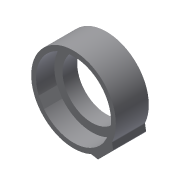
# Autodesk Inventor part: cellSTORM_objective_thread
Saved by Autodesk Inventor 2019 (Build 230136000, 136)
## iProperties
Created: 2019-10-25
Part Number: cellSTORM_objective_thread
Material: Generic
Document SubType Name: Modeling
Designer: marsikovabarbora
Density: 1 g/cm^3
Appearance: Default
Author: marsikovabarbora
Autodesk Inventor part; units mm, degrees
ref_plane "YZ Plane" through (0, 0, 0) normal (1, 0, 0) x (0, 1, 0)
ref_plane "XZ Plane" through (0, 0, 0) normal (0, 1, 0) x (-1, 0, 0)
ref_plane "XY Plane" through (0, 0, 0) normal (0, 0, 1) x (1, 0, 0)
sketch "Sketch1" plane through (0, 0, 0) normal (0, 0, 1) x (1, 0, 0)
  line L0 (9.6801, -14.008) -> (7.2052, -11.5331) construction
  line L1 (7.2052, -11.5331) -> (11.5893, -7.1491) construction
  line L2 (11.5893, -7.1491) -> (14.0642, -9.6239) construction
  line L3 (14.0642, -9.6239) -> (9.6801, -14.008) construction
  arc A0 (12.6369, -4.7496) -> (4.7496, -12.6369) centre (0, 0) ccw construction
  line L4 (10.9298, -3.0424) -> (12.6369, -4.7496) construction
  line L5 (11.6618, -4.6122) -> (10.9298, -3.0424) construction
  arc A1 (11.6618, -4.6122) -> (10.8551, -4.47) centre (11.2086, -4.8235) ccw construction
  line L6 (10.7915, -4.5335) -> (10.8551, -4.47) construction
  arc A2 (10.7915, -4.5335) -> (10.6527, -4.9738) centre (11.1451, -4.887) ccw construction
  line L7 (10.915, -6.4612) -> (10.6527, -4.9738) construction
  arc A3 (10.7761, -6.9016) -> (10.915, -6.4612) centre (10.4226, -6.548) ccw construction
  line L8 (6.9016, -10.7761) -> (10.7761, -6.9016) construction
  arc A4 (6.4612, -10.915) -> (6.9016, -10.7761) centre (6.548, -10.4226) ccw construction
  line L9 (6.4612, -10.915) -> (4.9738, -10.6527) construction
  arc A5 (4.9738, -10.6527) -> (4.5335, -10.7915) centre (4.887, -11.1451) ccw construction
  line L10 (4.5335, -10.7915) -> (4.47, -10.8551) construction
  arc A6 (4.47, -10.8551) -> (4.6122, -11.6618) centre (4.8235, -11.2086) ccw construction
  line L11 (4.6122, -11.6618) -> (3.0424, -10.9298) construction
  line L12 (3.0424, -10.9298) -> (4.7496, -12.6369) construction
  line L13 (-1.7167, -14.6498) -> (-1.7167, -17.5) construction
  line L14 (-1.7167, -17.5) -> (1.7167, -17.5) construction
  line L15 (1.7167, -14.6498) -> (1.7167, -17.5) construction
  arc A7 (1.7167, -14.6498) -> (6.9595, -13.0049) centre (0, 0) ccw construction
  arc A8 (6.9595, -13.0049) -> (8.2728, -15.1789) centre (8.2994, -13.6792) ccw construction
  line L16 (8.2728, -15.1789) -> (7.6816, -15.1684) construction
  arc A9 (8.5249, -17.8901) -> (7.6816, -15.1684) centre (7.655, -16.6682) ccw construction
  line L17 (8.5249, -17.8901) -> (13.5161, -14.3366) construction
  line L18 (13.5161, -14.3366) -> (13.5161, -12.2823) construction
  line L19 (13.5161, -12.2823) -> (14.6168, -12.2823) construction
  line L20 (14.6168, -12.2823) -> (14.6168, -1.9776) construction
  arc A10 (14.6168, -1.9776) -> (1.7167, 14.6498) centre (0, 0) ccw construction
  line L21 (1.7167, 14.6498) -> (1.7167, 17.5) construction
  line L22 (-1.7167, 17.5) -> (1.7167, 17.5) construction
  line L23 (-1.7167, 14.6498) -> (-1.7167, 17.5) construction
  arc A11 (-1.7167, 14.6498) -> (-14.2817, -3.6872) centre (0, 0) ccw construction
  line L24 (-14.2817, -3.6872) -> (-15.4135, -5.7935) construction
  arc A12 (-15.4135, -5.7935) -> (-14.5984, -8.502) centre (-13.6517, -6.7402) ccw construction
  line L25 (-14.5984, -8.502) -> (-9.6326, -11.1703) construction
  arc A13 (-9.6326, -11.1703) -> (-1.7167, -14.6498) centre (0, 0) ccw construction
  line L26 (-24.6, 24.6) -> (25.2, -25.2) construction
  line L27 (25.2, 24.6) -> (-24.6, -25.2) construction
  arc A14 (-1.4283, 10.15) -> (-9.5043, -3.8381) centre (0, 0) ccw
  circle A15 centre (0, 0) radius 10.1 construction
  line L28 (-1.4283, 10.15) -> (1.4283, 10.15)
  line L29 (-8.076, -6.3119) -> (-9.5043, -3.8381)
  line L30 (9.5043, -3.8381) -> (8.076, -6.3119)
  arc A16 (1.4283, 10.15) -> (-1.4283, 10.15) centre (0, 0) ccw
  arc A17 (9.5043, -3.8381) -> (1.4283, 10.15) centre (0, 0) ccw
  arc A18 (8.076, -6.3119) -> (9.5043, -3.8381) centre (0, 0) ccw
  arc A19 (-8.076, -6.3119) -> (8.076, -6.3119) centre (0, 0) ccw
  arc A20 (-9.5043, -3.8381) -> (-8.076, -6.3119) centre (0, 0) ccw
  arc A21 (10.7054, -6.8309) -> (10.8165, -6.4786) centre (10.4226, -6.548) ccw
  line L31 (10.8165, -6.4786) -> (10.5542, -4.9912)
  arc A22 (10.7208, -4.4628) -> (10.5956, -4.6461) centre (11.1451, -4.887) ccw construction
  line L32 (10.7208, -4.4628) -> (10.7844, -4.3992) construction
  arc A23 (11.7601, -5.0598) -> (10.7844, -4.3992) centre (11.2086, -4.8235) ccw construction
  line L33 (11.7601, -5.0598) -> (10.5994, -2.5707) construction
  line L34 (10.5994, -2.5707) -> (12.5972, -4.5684) construction
  arc A24 (12.5972, -4.5684) -> (4.5684, -12.5972) centre (0, 0) ccw construction
  line L35 (4.5684, -12.5972) -> (2.5707, -10.5994) construction
  line L36 (2.5707, -10.5994) -> (4.2491, -11.3821) construction
  arc A25 (4.3992, -10.7844) -> (4.2491, -11.3821) centre (4.8235, -11.2086) ccw construction
  line L37 (4.3992, -10.7844) -> (4.4628, -10.7208) construction
  arc A26 (4.9912, -10.5542) -> (4.6461, -10.5956) centre (4.887, -11.1451) ccw
  line L38 (4.9912, -10.5542) -> (6.4786, -10.8165)
  arc A27 (6.4786, -10.8165) -> (6.8309, -10.7054) centre (6.548, -10.4226) ccw
  line L39 (6.8309, -10.7054) -> (10.7054, -6.8309)
  circle A28 centre (0, 0) radius 11.5695
  arc A29 (4.6461, -10.5956) -> (4.4628, -10.7208) centre (4.887, -11.1451) ccw construction
  arc A30 (10.5956, -4.6461) -> (10.5542, -4.9912) centre (11.1451, -4.887) ccw
  dimension "d4" = 20.2
  dimension "d5" = 10.15
  dimension "d6" = 20.5
  dimension "d9" = 360
  dimension "d11" = 0.1
  constraints: 32 point on circle, 24 end point, 17 centre point, 4 tangent, 3 coincident, 1 horizontal, 21 other
  measures "d4" diameter of A15
  measures "d5" distance from line of L28 point (0, 0)
  measures "d6" diameter of A14
  measures "d11" distance between parallel lines of L8 L39
extrude "Extrusion1" add sketch "Sketch1" against normal blind 5 contours A16 L28 | L29 A20 | A18 L30 | L39 A27 L38 A26 A28 A30 L31 A21 | A28
sketch "Sketch3" plane through (0, 0, -5) normal (0, 0, -1) x (-1, 0, 0)
  line L0 (9.5043, -3.8381) -> (8.076, -6.3119) projected
  arc A0 (-8.076, -6.3119) -> (8.076, -6.3119) centre (0, 0) ccw projected
  line L1 (-8.076, -6.3119) -> (-9.5043, -3.8381) projected
  arc A1 (-1.4283, 10.15) -> (-9.5043, -3.8381) centre (0, 0) ccw projected
  line L2 (-1.4283, 10.15) -> (1.4283, 10.15) projected
  arc A2 (9.5043, -3.8381) -> (1.4283, 10.15) centre (0, 0) ccw projected
  arc A3 (-10.8165, -6.4786) -> (-10.7054, -6.8309) centre (-10.4226, -6.548) ccw projected
  line L3 (-10.7054, -6.8309) -> (-6.8309, -10.7054) projected
  arc A4 (-6.8309, -10.7054) -> (-6.4786, -10.8165) centre (-6.548, -10.4226) ccw projected
  line L4 (-6.4786, -10.8165) -> (-4.9912, -10.5542) projected
  arc A5 (-4.6461, -10.5956) -> (-4.9912, -10.5542) centre (-4.887, -11.1451) ccw projected
  arc A6 (-4.6461, -10.5956) -> (-10.5956, -4.6461) centre (0, 0) ccw projected
  arc A7 (-10.5542, -4.9912) -> (-10.5956, -4.6461) centre (-11.1451, -4.887) ccw projected
  line L5 (-10.5542, -4.9912) -> (-10.8165, -6.4786) projected
  circle A8 centre (0, 0) radius 8
  circle A9 centre (0, 0) radius 10.25
  dimension "d17" = 16
  constraints: 2 centre point, 2 coincident, 1 concentric
  measures "d17" diameter of A8
extrude "Extrusion3" add sketch "Sketch3" along normal blind 4 contours A9 L0 | L0 A0 L1 A1 L2 A2 | A9 L1 | L2 A9 | L5 A7 A6 A5 L4 A4 L3 A3
sketch "Sketch4" plane through (6.8309, -10.7054, 0) normal (0.7071068, -0.7071068, 0) x (0, 0, -1)
  line L0 (0, 0) -> (0, 5.4794) construction
  line L1 (0, 0) -> (9, 0) construction
  line L2 (9, 5.4794) -> (9, 0) construction
  line L3 (0, 5.4794) -> (9, 5.4794) construction
  line L4 (0, 2.7397) -> (9, 2.7397) construction
  circle A0 centre (7.2, 2.7397) radius 1.4
  dimension "d20" = 2.8
  dimension "d21" = 1.8
  constraints: 2 end point, 1 centre point, 1 midpoint, 1 point on line
  measures "d20" diameter of A0
  measures "d21" distance from line of L2 A0.centre
extrude "Extrusion4" cut sketch "Sketch4" against normal up to surface round surface about axis through (0, 0, -5) along (0, 0, -1) radius 8 far side no
body "Solid1"
